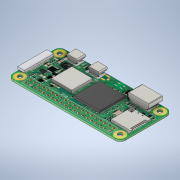
# Autodesk Inventor part: RPI_zero_2
Saved by Autodesk Inventor 2022.2 (Build 262287010, 287A)
## iProperties
Created: 2022-04-07
Part Number: RPI_zero_2
Material: 일반
Document SubType Name: Modeling
Designer: dbstj
Density: 1 g/cm^3
Appearance: 기본값
Mass: 3.14189 g
Surface Area: 46.9746 cm^2
Volume: 3.14189 cm^3
Author: dbstj
Autodesk Inventor part; units mm, degrees
ref_plane "YZ Plane" through (0, 0, 0) normal (1, 0, 0) x (0, 1, 0)
ref_plane "XZ Plane" through (0, 0, 0) normal (0, 1, 0) x (-1, 0, 0)
ref_plane "XY Plane" through (0, 0, 0) normal (0, 0, 1) x (1, 0, 0)
sketch "스케치1" plane through (0, 0, 0) normal (0, 0, 1) x (1, 0, 0)
  line L0 (-32.5, -15) -> (32.5, -15)
  line L1 (32.5, -15) -> (32.5, 15)
  line L2 (32.5, 15) -> (-32.5, 15)
  line L3 (-32.5, 15) -> (-32.5, -15)
  line L4 (-32.5, -15) -> (32.5, 15) construction
  line L5 (32.5, -15) -> (-32.5, 15) construction
  line L6 (-29, -11.5) -> (29, -11.5)
  line L7 (29, -11.5) -> (29, 11.5)
  line L8 (29, 11.5) -> (-29, 11.5)
  line L9 (-29, 11.5) -> (-29, -11.5)
  line L10 (-29, -11.5) -> (29, 11.5) construction
  line L11 (29, -11.5) -> (-29, 11.5) construction
  circle A0 centre (29, 11.5) radius 1.25
  circle A1 centre (29, -11.5) radius 1.25
  circle A2 centre (-29, -11.5) radius 1.25
  circle A3 centre (-29, 11.5) radius 1.25
  point P0 (0, 0)
  dimension "d0" = 65
  dimension "d1" = 30
  dimension "d2" = 58
  dimension "d3" = 23
  dimension "d4" = 2.5
  dimension "d5" = 2.5
  dimension "d6" = 2.5
  dimension "d7" = 2.5
  constraints: 24 end point, 4 centre point, 4 coincident, 4 midpoint, 4 parallel, 2 horizontal, 2 perpendicular
  measures "d0" distance of L2.end L1.end
  measures "d1" distance of L1.end L0.end
  measures "d2" distance of L8.end L7.end
  measures "d3" distance of L7.end L6.end
  measures "d4" diameter of A0
  measures "d5" diameter of A1
  measures "d6" diameter of A2
  measures "d7" diameter of A3
extrude "돌출1" add sketch "스케치1" along normal blind 1.1 contours L3 L2 L1 L0 | A2 L9 A3 L8 A0 L7 A1 L6
fillet "모깎기1" radius 3 4 edges at (32.5, 15, 0.55) (32.5, -15, 0.55) (-32.5, 15, 0.55) (-32.5, -15, 0.55)
sketch "스케치2" plane through (0, 0, 0) normal (0, 0, -1) x (-1, 0, 0)
  line L0 (33.5, 8.5) -> (29.5, 8.5)
  line L1 (29.5, 8.5) -> (29.5, -8.5)
  line L2 (29.5, -8.5) -> (33.5, -8.5)
  line L3 (33.5, -8.5) -> (33.5, 8.5)
  line L4 (32.5, 12) -> (32.5, -12) projected
  line L5 (-31.5, 8) -> (-20, 8)
  line L6 (-20, 8) -> (-20, -4)
  line L7 (-20, -4) -> (-31.5, -4)
  line L8 (-31.5, -4) -> (-31.5, 8)
  line L9 (-29.5, 15) -> (29.5, 15) projected
  line L10 (-32.5, -12) -> (-32.5, 12) projected
  line L11 (2.5, -8) -> (-12.5, -8)
  line L12 (-12.5, -8) -> (-12.5, 7)
  line L13 (-12.5, 7) -> (2.5, 7)
  line L14 (2.5, 7) -> (2.5, -8)
  point P0 (0, 0)
  point P1 (32.5, -8.5)
  point P2 (32.5, 8.5)
  dimension "d11" = 4
  dimension "d12" = 17
  dimension "d13" = 8.5
  dimension "d14" = 1
  dimension "d15" = 11.5
  dimension "d16" = 12
  dimension "d17" = 7
  dimension "d18" = 1
  dimension "d19" = 15
  dimension "d20" = 15
  dimension "d21" = 30
  dimension "d22" = 8
  constraints: 24 end point, 6 parallel, 3 horizontal, 3 perpendicular
  measures "d11" distance of L2.end L1.end
  measures "d12" distance of L1.end L0.end
  measures "d13" distance from line of point (0, 0) L2
  measures "d14" distance between parallel lines of L4 L3
  measures "d15" distance of L6.end L7.end
  measures "d16" distance of L5.end L6.end
  measures "d17" distance between parallel lines of L9 L5
  measures "d18" distance between parallel lines of L10 L8
  measures "d19" distance of L12.end L13.end
  measures "d20" distance of L11.end L12.end
  measures "d21" distance between parallel lines of L4 L14
  measures "d22" distance between parallel lines of L9 L13
extrude "돌출2" add sketch "스케치2" along normal blind 1.2
sketch "스케치3" plane through (0, 0, -1.2) normal (0, 0, -1) x (-1, 0, 0)
  line L0 (-31.5, -4) -> (-31.5, 8) projected
  line L1 (-31.5, 6.7292) -> (-30.1918, 6.7292)
  line L2 (-30.1918, 6.7292) -> (-30.1918, -1.7945)
  line L3 (-30.1918, -1.7945) -> (-31.5, -1.7945)
  line L4 (-31.5, -1.7945) -> (-31.5, 6.7292)
  point P0 (0, 0)
  constraints: 8 end point, 2 parallel, 1 horizontal, 1 perpendicular, 1 point on line
extrude "돌출3" cut sketch "스케치3" against normal blind 1.2
sketch "스케치4" plane through (0, 0, 0) normal (0, 0, -1) x (-1, 0, 0)
  line L0 (17.5, 5) -> (5.5, 5)
  line L1 (5.5, 5) -> (5.5, -7)
  line L2 (5.5, -7) -> (17.5, -7)
  line L3 (17.5, -7) -> (17.5, 5)
  line L4 (-29.5, 15) -> (29.5, 15) projected
  line L5 (2.5, -8) -> (2.5, 7) projected
  point P0 (0, 0)
  dimension "d27" = 12
  dimension "d28" = 12
  dimension "d29" = 10
  dimension "d30" = 3
  constraints: 8 end point, 2 parallel, 1 horizontal, 1 perpendicular
  measures "d27" distance of L2.end L1.end
  measures "d28" distance of L1.end L0.end
  measures "d29" distance between parallel lines of L4 L0
  measures "d30" distance between parallel lines of L5 L1
extrude "돌출4" add sketch "스케치4" along normal blind 1.5
sketch "스케치5" plane through (0, 0, 0) normal (0, 0, -1) x (-1, 0, 0)
  line L0 (25, -11) -> (18, -11)
  line L1 (18, -11) -> (18, -16)
  line L2 (18, -16) -> (25, -16)
  line L3 (25, -16) -> (25, -11)
  line L4 (12.4, -11) -> (5.4, -11)
  line L5 (5.4, -11) -> (5.4, -16)
  line L6 (5.4, -16) -> (12.4, -16)
  line L7 (12.4, -16) -> (12.4, -11)
  line L8 (29.5, -15) -> (-29.5, -15) projected
  line L9 (32.5, -8.5) -> (32.5, -12) projected
  line L10 (-32.5, -12) -> (-32.5, 12) projected
  point P0 (0, 0)
  point P1 (8.9, -16)
  point P2 (21.5, -16)
  dimension "d33" = 7
  dimension "d34" = 5
  dimension "d35" = 7
  dimension "d36" = 5
  dimension "d37" = 1
  dimension "d312" = 41.4
  dimension "d313" = 54
  constraints: 16 end point, 4 parallel, 2 horizontal, 2 midpoint, 2 perpendicular, 1 point on line
  measures "d33" distance of L2.end L1.end
  measures "d34" distance of L1.end L0.end
  measures "d35" distance of L6.end L5.end
  measures "d36" distance of L5.end L4.end
  measures "d37" distance between parallel lines of L8 L2
  measures "d312" distance from line of L10 point (8.9, -16)
  measures "d313" distance from line of L10 point (21.5, -16)
extrude "돌출5" add sketch "스케치5" along normal blind 2.5
sketch "스케치6" plane through (-25, -16, 0) normal (0, -1, 0) x (1, 0, 0)
  line L0 (7, 0) -> (0, 0) projected
  line L1 (0, 0) -> (1.5, 0)
  line L2 (0, -2.5) -> (7, -2.5) projected
  line L3 (1.5, 0) -> (0, -2.5)
  line L4 (0, 0) -> (0, -2.5) projected
  line L5 (0, -2.5) -> (0, 0)
  line L6 (7, 0) -> (12.6, 0) projected
  line L7 (7, 0) -> (5.5, 0)
  line L8 (5.5, 0) -> (7, -2.5)
  line L9 (7, -2.5) -> (7, 0)
  line L10 (12.6, 0) -> (14.1, 0)
  line L11 (12.6, 0) -> (19.6, 0) projected
  line L12 (19.6, -2.5) -> (12.6, -2.5) projected
  line L13 (14.1, 0) -> (12.6, -2.5)
  line L14 (12.6, -2.5) -> (12.6, 0)
  line L15 (19.6, 0) -> (18.1, 0)
  line L16 (19.6, 0) -> (19.6, -2.5) projected
  line L17 (18.1, 0) -> (19.6, -2.5)
  line L18 (19.6, -2.5) -> (19.6, 0)
  line L19 (19.5, 0) -> (7.5, 0) projected
  point P0 (25, 0)
  dimension "d42" = 1.5
  dimension "d43" = 1.5
  dimension "d44" = 1.5
  dimension "d45" = 1.5
  constraints: 24 end point, 5 point on line, 3 perpendicular, 1 collinear
  measures "d42" distance of L0.end L1.end
  measures "d43" distance of L0.start L7.end
  measures "d44" distance of L10.start L10.end
  measures "d45" distance of L11.end L15.end
extrude "돌출6" cut sketch "스케치6" against normal blind 5 contours L9 L8 L0 | L3 L4 L0 | L10 L13 L14 | L11 L16 L17
sketch "스케치7" plane through (0, 0, 0) normal (0, 0, -1) x (-1, 0, 0)
  line L0 (-26.1, -16) -> (-14.1, -16)
  line L1 (-14.1, -16) -> (-14.1, -8)
  line L2 (-14.1, -8) -> (-26.1, -8)
  line L3 (-26.1, -8) -> (-26.1, -16)
  line L4 (6.9, -15) -> (-29.5, -15) projected
  line L5 (-32.5, -12) -> (-32.5, 12) projected
  point P0 (0, 0)
  point P1 (-20.1, -16)
  dimension "d48" = 12
  dimension "d49" = 8
  dimension "d50" = 1
  dimension "d315" = 12.4
  constraints: 8 end point, 2 parallel, 1 horizontal, 1 midpoint, 1 perpendicular
  measures "d48" distance of L2.end L1.end
  measures "d49" distance of L1.end L0.end
  measures "d50" distance between parallel lines of L4 L0
  measures "d315" distance from line of L5 point (-20.1, -16)
extrude "돌출7" add sketch "스케치7" along normal blind 4
sketch "스케치8" plane through (14.1, -16, 0) normal (0, -1, 0) x (1, 0, 0)
  line L0 (0, 0) -> (12, 0) projected
  line L1 (0, 0) -> (2, 0)
  line L2 (2, 0) -> (0, -1.6782)
  line L3 (0, 0) -> (0, -4)
  line L4 (0, -3.8) -> (0.2, -4)
  line L5 (0, -4) -> (12, -4) projected
  line L6 (2, -4) -> (0, -4)
  line L7 (0, -4) -> (0, 0)
  line L8 (12, 0) -> (12, -4)
  line L9 (12, 0) -> (10, 0)
  line L10 (10, 0) -> (12, -1.6782)
  line L11 (12, -3.8) -> (11.8, -4)
  line L12 (10, -4) -> (12, -4)
  line L13 (12, -4) -> (12, 0)
  line L14 (12, 0) -> (12, -4) projected
  line L15 (12, -4) -> (0, -4) projected
  line L16 (0, 0) -> (0, -4) projected
  point P0 (-14.1, 0)
  point P1 (12, -1.6782)
  dimension "d54" = 2
  dimension "d55" = 40
  dimension "d56" = 2
  dimension "d306" = 0.2
  dimension "d307" = 0.2
  dimension "d308" = 40
  dimension "d309" = 0.2
  dimension "d310" = 0.2
  constraints: 24 end point, 7 point on line, 1 horizontal, 1 parallel, 1 perpendicular
  measures "d54" distance of L0.start L1.end
  measures "d55" angle of L1 L2
  measures "d56" distance of L0.end L9.end
  measures "d306" distance from line of L11.start L5
  measures "d307" distance of L11.end L5.end
  measures "d308" angle of L9 L10
  measures "d309" distance of L3.end L4.start
  measures "d310" distance of L4.end L3.end
extrude "돌출8" cut sketch "스케치8" against normal blind 8 contours L0 L2 L3 | L0 L8 L10 | L4 L5 L3 | L8 L5 L11
fillet "모깎기2" radius 0.5 12 edges at (25.9, -12, -4) (14.3, -12, -4) (-5.4, -13.5, -2.5) (-12.4, -13.5, -2.5) (-18, -13.5, -2.5) (-25, -13.5, -2.5) (16.1, -15.5, 0) (24.1, -15.5, 0) (-6.9, -15.5, 0) (-19.5, -15.5, 0) (-23.5, -15.5, 0) (-10.9, -15.5, 0)
sketch "스케치12" plane through (16.282, -16, 0) normal (0, -1, 0) x (1, 0, 0)
  arc A0 (7.9574, -0.117) -> (7.636, 0) centre (7.636, -0.5) ccw projected
  line L0 (7.636, 0) -> (0, 0) projected
  arc A1 (0, 0) -> (-0.3214, -0.117) centre (0, -0.5) ccw projected
  line L1 (-0.3214, -0.117) -> (-2.182, -1.6782) projected
  line L2 (-2.182, -3.8) -> (-2.1284, -3.8536) projected
  arc A2 (-2.1284, -3.8536) -> (-1.7749, -4) centre (-1.7749, -3.5) ccw projected
  line L3 (9.4109, -4) -> (-1.7749, -4) projected
  arc A3 (9.4109, -4) -> (9.7645, -3.8536) centre (9.4109, -3.5) ccw projected
  line L4 (9.7645, -3.8536) -> (9.818, -3.8) projected
  line L5 (9.818, -1.6782) -> (7.9574, -0.117) projected
  line L6 (-1.9335, -3.4828) -> (-2.4355, -2.9808)
  line L7 (-2.4098, -2.3915) -> (-0.1479, -0.4936)
  line L8 (0.1092, -0.4) -> (7.5268, -0.4)
  line L9 (7.784, -0.4936) -> (10.0458, -2.3915)
  line L10 (10.0716, -2.9808) -> (9.5695, -3.4828)
  line L11 (9.2866, -3.6) -> (-1.6506, -3.6)
  arc A4 (-2.4098, -2.3915) -> (-2.4355, -2.9808) centre (-2.1527, -2.6979) ccw
  arc A5 (-1.9335, -3.4828) -> (-1.6506, -3.6) centre (-1.6506, -3.2) ccw
  arc A6 (10.0716, -2.9808) -> (10.0458, -2.3915) centre (9.7887, -2.6979) ccw
  arc A7 (0.1092, -0.4) -> (-0.1479, -0.4936) centre (0.1092, -0.8) ccw
  arc A8 (7.784, -0.4936) -> (7.5268, -0.4) centre (7.5268, -0.8) ccw
  arc A9 (9.2866, -3.6) -> (9.5695, -3.4828) centre (9.2866, -3.2) ccw
  line L12 (-2.182, -1.6782) -> (-2.182, -3.8) projected
  line L13 (9.818, -1.6782) -> (9.818, -3.8) projected
  arc A10 (-1.782, -3.5997) -> (-1.7749, -3.6) centre (-1.7749, -3.5) ccw
  line L14 (-1.782, -3.5997) -> (-1.782, -1.8647)
  line L15 (-1.782, -1.8647) -> (-0.0643, -0.4234)
  arc A11 (0, -0.4) -> (-0.0643, -0.4234) centre (0, -0.5) ccw
  line L16 (0, -0.4) -> (7.636, -0.4)
  arc A12 (7.7003, -0.4234) -> (7.636, -0.4) centre (7.636, -0.5) ccw
  line L17 (7.7003, -0.4234) -> (9.418, -1.8647)
  line L18 (9.418, -1.8647) -> (9.418, -3.5997)
  arc A13 (9.4109, -3.6) -> (9.418, -3.5997) centre (9.4109, -3.5) ccw
  line L19 (9.4109, -3.6) -> (-1.7749, -3.6)
  point P0 (-16.282, 0)
  point P1 (9.418, -3.5778)
  point P2 (9.418, -1.8647)
  point P3 (-1.782, -1.8647)
  point P4 (-1.782, -3.5778)
  dimension "d85" = 0.4
  dimension "d86" = 0.4
  dimension "d311" = 0.4
  constraints: 24 end point, 20 point on circle, 12 tangent, 10 centre point, 4 equal radius, 14 other
  measures "d85" distance between parallel lines of L3 L11
  measures "d86" radius of A4
  measures "d311" distance between parallel lines of L3 L19
extrude "돌출10" cut sketch "스케치12" against normal blind 6 contours L18 A9 L11 A5 L14 L7 A7 L8 A8 L9
sketch "스케치13" plane through (-10.6169, -16, 0) normal (0, -1, 0) x (1, 0, 0)
  arc A0 (0, 0) -> (-0.4287, -0.2428) centre (0, -0.5) ccw projected
  line L0 (-0.4287, -0.2428) -> (-1.3287, -1.7428) projected
  arc A1 (-1.3287, -1.7428) -> (-0.9, -2.5) centre (-0.9, -2) ccw projected
  line L1 (4.3338, -2.5) -> (-0.9, -2.5) projected
  arc A2 (4.3338, -2.5) -> (4.7626, -1.7428) centre (4.3338, -2) ccw projected
  line L2 (4.7626, -1.7428) -> (3.8626, -0.2428) projected
  arc A3 (3.8626, -0.2428) -> (3.4338, 0) centre (3.4338, -0.5) ccw projected
  line L3 (3.4338, 0) -> (0, 0) projected
  arc A4 (-12.6, 0) -> (-13.0287, -0.2428) centre (-12.6, -0.5) ccw projected
  line L4 (-13.0287, -0.2428) -> (-13.9287, -1.7428) projected
  arc A5 (-13.9287, -1.7428) -> (-13.5, -2.5) centre (-13.5, -2) ccw projected
  line L5 (-8.2662, -2.5) -> (-13.5, -2.5) projected
  arc A6 (-8.2662, -2.5) -> (-7.8374, -1.7428) centre (-8.2662, -2) ccw projected
  line L6 (-7.8374, -1.7428) -> (-8.7374, -0.2428) projected
  arc A7 (-8.7374, -0.2428) -> (-9.1662, 0) centre (-9.1662, -0.5) ccw projected
  line L7 (-9.1662, 0) -> (-12.6, 0) projected
  arc A8 (-1.0715, -1.8971) -> (-0.9, -2.2) centre (-0.9, -2) ccw
  line L8 (-1.0715, -1.8971) -> (-0.1715, -0.3971)
  arc A9 (0, -0.3) -> (-0.1715, -0.3971) centre (0, -0.5) ccw
  line L9 (0, -0.3) -> (3.4338, -0.3)
  arc A10 (3.6053, -0.3971) -> (3.4338, -0.3) centre (3.4338, -0.5) ccw
  line L10 (3.6053, -0.3971) -> (4.5053, -1.8971)
  arc A11 (4.3338, -2.2) -> (4.5053, -1.8971) centre (4.3338, -2) ccw
  line L11 (4.3338, -2.2) -> (-0.9, -2.2)
  arc A12 (-13.6715, -1.8971) -> (-13.5, -2.2) centre (-13.5, -2) ccw
  line L12 (-13.6715, -1.8971) -> (-12.7715, -0.3971)
  arc A13 (-12.6, -0.3) -> (-12.7715, -0.3971) centre (-12.6, -0.5) ccw
  line L13 (-12.6, -0.3) -> (-9.1662, -0.3)
  arc A14 (-8.9947, -0.3971) -> (-9.1662, -0.3) centre (-9.1662, -0.5) ccw
  line L14 (-8.9947, -0.3971) -> (-8.0947, -1.8971)
  arc A15 (-8.2662, -2.2) -> (-8.0947, -1.8971) centre (-8.2662, -2) ccw
  line L15 (-8.2662, -2.2) -> (-13.5, -2.2)
  point P0 (10.6169, 0)
  dimension "d11" = 4
  dimension "d12" = 17
  dimension "d13" = 8.5
  dimension "d14" = 1
  dimension "d89" = 0.3
  dimension "d90" = 0.3
  constraints: 16 end point, 16 point on circle, 8 centre point, 14 other
  measures "d89" distance between parallel lines of L1 L11
  measures "d90" distance between parallel lines of L5 L15
extrude "돌출11" cut sketch "스케치13" against normal blind 4 contours L8 A9 L9 A10 L10 A11 L11 A8 | L12 A13 L13 A14 L14 A15 L15 A12
sketch "스케치14" plane through (0, 0, 0) normal (0, 0, -1) x (-1, 0, 0)
  line L0 (-29.5, 15) -> (29.5, 15) projected
  circle A0 centre (-29, 11.5) radius 1.25 projected
  point P0 (0, 0)
  point P1 (24.13, 12.77)
  point P2 (24.13, 10.23)
  point P3 (21.59, 10.23)
  point P4 (19.05, 12.77)
  point P5 (16.51, 12.77)
  point P6 (13.97, 12.77)
  point P7 (11.43, 12.77)
  point P8 (8.89, 12.77)
  point P9 (6.35, 12.77)
  point P10 (3.81, 12.77)
  point P11 (1.27, 12.77)
  point P12 (-1.27, 12.77)
  point P13 (-3.81, 12.77)
  point P14 (-6.35, 12.77)
  point P15 (-8.89, 12.77)
  point P16 (-11.43, 12.77)
  point P17 (-13.97, 12.77)
  point P18 (-16.51, 12.77)
  point P19 (-19.05, 12.77)
  point P20 (-21.59, 12.77)
  point P21 (19.05, 10.23)
  point P22 (16.51, 10.23)
  point P23 (13.97, 10.23)
  point P24 (11.43, 10.23)
  point P25 (8.89, 10.23)
  point P26 (6.35, 10.23)
  point P27 (3.81, 10.23)
  point P28 (1.27, 10.23)
  point P29 (-1.27, 10.23)
  point P30 (-3.81, 10.23)
  point P31 (-6.35, 10.23)
  point P32 (-8.89, 10.23)
  point P33 (-11.43, 10.23)
  point P34 (-13.97, 10.23)
  point P35 (-16.51, 10.23)
  point P36 (-19.05, 10.23)
  point P37 (-21.59, 10.23)
  point P38 (-24.13, 10.23)
  point P39 (-24.13, 12.77)
  point P40 (21.59, 12.77)
  dimension "d94" = 2.54
  dimension "d95" = 2.54
  dimension "d96" = 2.54
  dimension "d97" = 2.54
  dimension "d98" = 2.54
  dimension "d99" = 2.54
  dimension "d100" = 2.54
  dimension "d101" = 2.54
  dimension "d102" = 2.54
  dimension "d103" = 2.54
  dimension "d104" = 2.54
  dimension "d105" = 2.54
  dimension "d106" = 2.54
  dimension "d107" = 2.54
  dimension "d108" = 2.54
  dimension "d109" = 2.54
  dimension "d112" = 2.54
  dimension "d114" = 2.23
  dimension "d317" = 2.54
  dimension "d318" = 2.54
  dimension "d319" = 2.54
  dimension "d320" = 27.73
  constraints: 38 horizontal alignment, 20 vertical alignment
  measures "d94" distance of point (-21.59, 12.77) point (-19.05, 12.77)
  measures "d95" distance of point (-16.51, 12.77) point (-19.05, 12.77)
  measures "d96" distance of point (-13.97, 12.77) point (-16.51, 12.77)
  measures "d97" distance of point (-11.43, 12.77) point (-13.97, 12.77)
  measures "d98" distance of point (-8.89, 12.77) point (-11.43, 12.77)
  measures "d99" distance of point (-6.35, 12.77) point (-8.89, 12.77)
  measures "d100" distance of point (-3.81, 12.77) point (-6.35, 12.77)
  measures "d101" distance of point (-1.27, 12.77) point (-3.81, 12.77)
  measures "d102" distance of point (1.27, 12.77) point (-1.27, 12.77)
  measures "d103" distance of point (3.81, 12.77) point (1.27, 12.77)
  measures "d104" distance of point (6.35, 12.77) point (3.81, 12.77)
  measures "d105" distance of point (8.89, 12.77) point (6.35, 12.77)
  measures "d106" distance of point (11.43, 12.77) point (8.89, 12.77)
  measures "d107" distance of point (13.97, 12.77) point (11.43, 12.77)
  measures "d108" distance of point (16.51, 12.77) point (13.97, 12.77)
  measures "d109" distance of point (19.05, 12.77) point (16.51, 12.77)
  measures "d112" distance of point (24.13, 12.77) point (24.13, 10.23)
  measures "d114" distance from line of L0 point (24.13, 12.77)
  measures "d317" distance of point (21.59, 12.77) point (19.05, 12.77)
  measures "d318" distance of point (24.13, 12.77) point (21.59, 12.77)
  measures "d319" distance of point (-21.59, 12.77) point (-24.13, 12.77)
  measures "d320" horizontal distance of point (-1.27, 12.77) A0.centre
hole "구멍3" at (-24.13, 12.77, 0) at (-24.13, 10.23, 0) at (-21.59, 10.23, 0) at (-19.05, 12.77, 0) at (-16.51, 12.77, 0) at (-13.97, 12.77, 0) at (-11.43, 12.77, 0) at (-8.89, 12.77, 0) at (-6.35, 12.77, 0) at (-3.81, 12.77, 0) at (-1.27, 12.77, 0) at (1.27, 12.77, 0) at (3.81, 12.77, 0) at (6.35, 12.77, 0) at (8.89, 12.77, 0) at (11.43, 12.77, 0) at (13.97, 12.77, 0) at (16.51, 12.77, 0) at (19.05, 12.77, 0) at (21.59, 12.77, 0) at (-19.05, 10.23, 0) at (-16.51, 10.23, 0) at (-13.97, 10.23, 0) at (-11.43, 10.23, 0) at (-8.89, 10.23, 0) at (-6.35, 10.23, 0) at (-3.81, 10.23, 0) at (-1.27, 10.23, 0) at (1.27, 10.23, 0) at (3.81, 10.23, 0) at (6.35, 10.23, 0) at (8.89, 10.23, 0) at (11.43, 10.23, 0) at (13.97, 10.23, 0) at (16.51, 10.23, 0) at (19.05, 10.23, 0) at (21.59, 10.23, 0) at (24.13, 10.23, 0) at (24.13, 12.77, 0) at (-21.59, 12.77, 0) direction (0, 0, 1) diameter 1 end through all
sketch "스케치17" plane through (32.5, -12, 0) normal (1, 0, 0) x (0, 0, -1)
  line L0 (0, 20.5) -> (0, 3.5) projected
  line L1 (0, 19.5) -> (1, 19.5)
  line L2 (1, 19.5) -> (1, 8.5)
  line L3 (1, 8.5) -> (0, 8.5)
  line L4 (0, 8.5) -> (0, 19.5)
  line L5 (0, 8) -> (1.2, 8) projected
  point P0 (0, 12)
  point P1 (0, 8.5)
  dimension "d238" = 1
  dimension "d239" = 11
  dimension "d240" = 0.5
  constraints: 8 end point, 2 parallel, 1 horizontal, 1 perpendicular, 1 point on line
  measures "d238" distance of L2.end L3.end
  measures "d239" distance of L1.end L2.end
  measures "d240" distance between parallel lines of L5 L3
extrude "돌출12" cut sketch "스케치17" against normal blind 12
sketch "스케치18" plane through (0, 0, -1.2) normal (0, 0, -1) x (-1, 0, 0)
  line L0 (-20.5, 7.5) -> (-20.5, -3.5) projected
  line L1 (-20.5, -3.5) -> (-22.5, -3.5)
  line L2 (-22.5, -3.5) -> (-22.5, -1.6212)
  line L3 (-22.5, -1.6212) -> (-20.5, -1.6212)
  line L4 (-20.5, -1.6212) -> (-20.5, -3.5)
  line L5 (-31.5, -3.5) -> (-20.5, -3.5) projected
  line L6 (-24.5, -3.5) -> (-25, -3.5)
  line L7 (-25, -3.5) -> (-25, -2.9865)
  line L8 (-25, -2.9865) -> (-24.5, -2.9865)
  line L9 (-24.5, -2.9865) -> (-24.5, -3.5)
  line L10 (-27, -3.5) -> (-27.5, -3.5)
  line L11 (-27.5, -3.5) -> (-27.5, -2.9865)
  line L12 (-27.5, -2.9865) -> (-27, -2.9865)
  line L13 (-27, -2.9865) -> (-27, -3.5)
  point P0 (0, 0)
  dimension "d245" = 2
  dimension "d246" = 2
  dimension "d247" = 2
  dimension "d248" = 0.5
  dimension "d249" = 0.5
  constraints: 24 end point, 6 parallel, 3 horizontal, 3 perpendicular, 3 point on line
  measures "d245" distance of L2.end L3.end
  measures "d246" distance between parallel lines of L2 L9
  measures "d247" distance between parallel lines of L13 L7
  measures "d248" distance of L7.end L8.end
  measures "d249" distance of L11.end L12.end
extrude "돌출13" cut sketch "스케치18" against normal up to surface (0.2 mm away)
sketch "스케치20" plane through (0, 0, 0) normal (0, 0, -1) x (-1, 0, 0)
  line L0 (-32.7551, 15.5771) -> (32.9909, 15.17) construction
  line L1 (32.9909, 15.17) -> (32.8001, -15.638) construction
  line L2 (32.8001, -15.638) -> (-32.9458, -15.2309) construction
  line L3 (-32.9458, -15.2309) -> (-32.7551, 15.5771) construction
  line L4 (-31.5, 7.5) -> (-31.5, 8) projected
  line L5 (-31.5, 8) -> (-20, 8) projected
  line L6 (-20, 8) -> (-20, -4) projected
  line L7 (-20, -4) -> (-31.5, -4) projected
  line L8 (-31.5, -4) -> (-31.5, -3.5) projected
  line L9 (-31.5, -3.5) -> (-20.5, -3.5) projected
  line L10 (-20.5, -3.5) -> (-20.5, 7.5) projected
  line L11 (-31.5, 7.5) -> (-20.5, 7.5) projected
  circle A0 centre (29, 11.5) radius 1.25 projected
  circle A1 centre (-29, 11.5) radius 1.25 projected
  circle A2 centre (-29, -11.5) radius 1.25 projected
  circle A3 centre (29, -11.5) radius 1.25 projected
  line L12 (2.5, 7) -> (2.5, -8) projected
  line L13 (2.5, -8) -> (-12.5, -8) projected
  line L14 (-12.5, -8) -> (-12.5, 7) projected
  line L15 (-12.5, 7) -> (2.5, 7) projected
  line L16 (-32.5, -12) -> (-32.5, 12) projected
  arc A4 (-32.5, -12) -> (-29.5, -15) centre (-29.5, -12) ccw projected
  line L17 (-24.1, -15) -> (-29.5, -15) projected
  line L18 (-24.1, -15) -> (-24.1, -8) projected
  line L19 (-24.1, -8) -> (-16.1, -8) projected
  line L20 (-16.1, -15) -> (-16.1, -8) projected
  line L21 (6.9, -15) -> (-16.1, -15) projected
  line L22 (6.9, -15) -> (6.9, -11) projected
  line L23 (6.9, -11) -> (10.9, -11) projected
  line L24 (10.9, -15) -> (10.9, -11) projected
  line L25 (19.5, -15) -> (10.9, -15) projected
  line L26 (19.5, -15) -> (19.5, -11) projected
  line L27 (19.5, -11) -> (23.5, -11) projected
  line L28 (23.5, -15) -> (23.5, -11) projected
  line L29 (29.5, -15) -> (23.5, -15) projected
  arc A5 (29.5, -15) -> (32.5, -12) centre (29.5, -12) ccw projected
  line L30 (32.5, -8.5) -> (32.5, -12) projected
  line L31 (32.5, -8.5) -> (29.5, -8.5) projected
  line L32 (29.5, -8.5) -> (29.5, 8.5) projected
  line L33 (29.5, 8.5) -> (32.5, 8.5) projected
  line L34 (32.5, 12) -> (32.5, 8.5) projected
  arc A6 (32.5, 12) -> (29.5, 15) centre (29.5, 12) ccw projected
  line L35 (-29.5, 15) -> (29.5, 15) projected
  arc A7 (-29.5, 15) -> (-32.5, 12) centre (-29.5, 12) ccw projected
  line L36 (5.5, 5) -> (17.5, 5) projected
  line L37 (17.5, 5) -> (17.5, -7) projected
  line L38 (17.5, -7) -> (5.5, -7) projected
  line L39 (5.5, -7) -> (5.5, 5) projected
  circle A8 centre (-24.13, 10.23) radius 0.5 projected
  circle A9 centre (-19.05, 10.23) radius 0.5 projected
  circle A10 centre (-13.97, 10.23) radius 0.5 projected
  circle A11 centre (-8.89, 10.23) radius 0.5 projected
  circle A12 centre (-3.81, 10.23) radius 0.5 projected
  circle A13 centre (1.27, 10.23) radius 0.5 projected
  circle A14 centre (6.35, 10.23) radius 0.5 projected
  circle A15 centre (11.43, 10.23) radius 0.5 projected
  circle A16 centre (16.51, 10.23) radius 0.5 projected
  circle A17 centre (-21.59, 12.77) radius 0.5 projected
  circle A18 centre (-16.51, 12.77) radius 0.5 projected
  circle A19 centre (-11.43, 12.77) radius 0.5 projected
  circle A20 centre (-6.35, 12.77) radius 0.5 projected
  circle A21 centre (-1.27, 12.77) radius 0.5 projected
  circle A22 centre (3.81, 12.77) radius 0.5 projected
  circle A23 centre (8.89, 12.77) radius 0.5 projected
  circle A24 centre (13.97, 12.77) radius 0.5 projected
  circle A25 centre (19.05, 12.77) radius 0.5 projected
  circle A26 centre (24.13, 10.23) radius 0.5 projected
  circle A27 centre (24.13, 12.77) radius 0.5 projected
  circle A28 centre (21.59, 10.23) radius 0.5 projected
  circle A29 centre (16.51, 12.77) radius 0.5 projected
  circle A30 centre (11.43, 12.77) radius 0.5 projected
  circle A31 centre (6.35, 12.77) radius 0.5 projected
  circle A32 centre (1.27, 12.77) radius 0.5 projected
  circle A33 centre (-3.81, 12.77) radius 0.5 projected
  circle A34 centre (-8.89, 12.77) radius 0.5 projected
  circle A35 centre (-13.97, 12.77) radius 0.5 projected
  circle A36 centre (-19.05, 12.77) radius 0.5 projected
  circle A37 centre (19.05, 10.23) radius 0.5 projected
  circle A38 centre (13.97, 10.23) radius 0.5 projected
  circle A39 centre (8.89, 10.23) radius 0.5 projected
  circle A40 centre (3.81, 10.23) radius 0.5 projected
  circle A41 centre (-1.27, 10.23) radius 0.5 projected
  circle A42 centre (-6.35, 10.23) radius 0.5 projected
  circle A43 centre (-11.43, 10.23) radius 0.5 projected
  circle A44 centre (-16.51, 10.23) radius 0.5 projected
  circle A45 centre (-21.59, 10.23) radius 0.5 projected
  point P0 (0, 0)
  constraints: 2 other
decal "전사3"
sketch "스케치21" plane through (0, 0, 1.1) normal (0, 0, 1) x (1, 0, 0)
  line L0 (-32.3589, 14.8407) -> (32.4304, 14.6694) construction
  line L1 (32.4304, 14.6694) -> (32.3526, -14.769) construction
  line L2 (32.3526, -14.769) -> (-32.4367, -14.5978) construction
  line L3 (-32.4367, -14.5978) -> (-32.3589, 14.8407) construction
  circle A0 centre (24.13, 12.77) radius 0.5 projected
  circle A1 centre (21.59, 10.23) radius 0.5 projected
  circle A2 centre (16.51, 10.23) radius 0.5 projected
  circle A3 centre (11.43, 10.23) radius 0.5 projected
  circle A4 centre (6.35, 10.23) radius 0.5 projected
  circle A5 centre (1.27, 10.23) radius 0.5 projected
  circle A6 centre (-3.81, 10.23) radius 0.5 projected
  circle A7 centre (-8.89, 10.23) radius 0.5 projected
  circle A8 centre (-13.97, 10.23) radius 0.5 projected
  circle A9 centre (-19.05, 10.23) radius 0.5 projected
  circle A10 centre (19.05, 12.77) radius 0.5 projected
  circle A11 centre (13.97, 12.77) radius 0.5 projected
  circle A12 centre (8.89, 12.77) radius 0.5 projected
  circle A13 centre (3.81, 12.77) radius 0.5 projected
  circle A14 centre (-1.27, 12.77) radius 0.5 projected
  circle A15 centre (-6.35, 12.77) radius 0.5 projected
  circle A16 centre (-11.43, 12.77) radius 0.5 projected
  circle A17 centre (-16.51, 12.77) radius 0.5 projected
  circle A18 centre (-21.59, 10.23) radius 0.5 projected
  circle A19 centre (-24.13, 12.77) radius 0.5 projected
  circle A20 centre (-24.13, 10.23) radius 0.5 projected
  circle A21 centre (-19.05, 12.77) radius 0.5 projected
  circle A22 centre (-13.97, 12.77) radius 0.5 projected
  circle A23 centre (-8.89, 12.77) radius 0.5 projected
  circle A24 centre (-3.81, 12.77) radius 0.5 projected
  circle A25 centre (1.27, 12.77) radius 0.5 projected
  circle A26 centre (6.35, 12.77) radius 0.5 projected
  circle A27 centre (11.43, 12.77) radius 0.5 projected
  circle A28 centre (16.51, 12.77) radius 0.5 projected
  circle A29 centre (21.59, 12.77) radius 0.5 projected
  circle A30 centre (-16.51, 10.23) radius 0.5 projected
  circle A31 centre (-11.43, 10.23) radius 0.5 projected
  circle A32 centre (-6.35, 10.23) radius 0.5 projected
  circle A33 centre (-1.27, 10.23) radius 0.5 projected
  circle A34 centre (3.81, 10.23) radius 0.5 projected
  circle A35 centre (8.89, 10.23) radius 0.5 projected
  circle A36 centre (13.97, 10.23) radius 0.5 projected
  circle A37 centre (19.05, 10.23) radius 0.5 projected
  circle A38 centre (24.13, 10.23) radius 0.5 projected
  circle A39 centre (-21.59, 12.77) radius 0.5 projected
  arc A40 (-32.5, -12) -> (-29.5, -15) centre (-29.5, -12) ccw projected
  line L4 (-29.5, -15) -> (29.5, -15) projected
  arc A41 (29.5, -15) -> (32.5, -12) centre (29.5, -12) ccw projected
  line L5 (32.5, -12) -> (32.5, 12) projected
  arc A42 (32.5, 12) -> (29.5, 15) centre (29.5, 12) ccw projected
  line L6 (29.5, 15) -> (-29.5, 15) projected
  arc A43 (-29.5, 15) -> (-32.5, 12) centre (-29.5, 12) ccw projected
  line L7 (-32.5, 12) -> (-32.5, -12) projected
  circle A44 centre (-29, -11.5) radius 1.25 projected
  circle A45 centre (29, -11.5) radius 1.25 projected
  circle A46 centre (29, 11.5) radius 1.25 projected
  circle A47 centre (-29, 11.5) radius 1.25 projected
  point P0 (0, 0)
  constraints: 2 other
decal "전사4"
equation "\"d13\" = 0.5 * d12"
equation "\"d94\" = d93"
equation "\"d95\" = d93"
equation "\"d96\" = d93"
equation "\"d97\" = d93"
equation "\"d98\" = d93"
equation "\"d99\" = d93"
equation "\"d100\" = d93"
equation "\"d101\" = d93"
equation "\"d102\" = d93"
equation "\"d103\" = d93"
equation "\"d104\" = d93"
equation "\"d105\" = d93"
equation "\"d106\" = d93"
equation "\"d107\" = d93"
equation "\"d108\" = d93"
equation "\"d109\" = d93"
equation "\"d317\" = d109"
equation "\"d318\" = d109"
equation "\"d319\" = d94"
equation "\"d93\" = 2.54"
